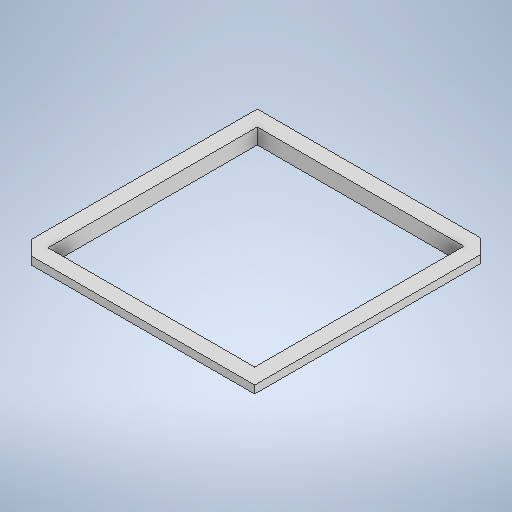
# Autodesk Inventor part: Installation Tool Collar
Saved by Autodesk Inventor 2025 (Build 290162000, 162)
## iProperties
Created: 2025-03-25
Part Number: Installation Tool Collar
Material: Generic
Document SubType Name: Modeling
Designer: Caleb Fangmeier
Density: 1 g/cm^3
Appearance: Default
Author: Caleb Fangmeier
Autodesk Inventor part; units mm, degrees
ref_plane "YZ Plane" through (0, 0, 0) normal (1, 0, 0) x (0, 1, 0)
ref_plane "XZ Plane" through (0, 0, 0) normal (0, 1, 0) x (-1, 0, 0)
ref_plane "XY Plane" through (0, 0, 0) normal (0, 0, 1) x (1, 0, 0)
sketch "Sketch1" plane through (0, 0, 0) normal (0, 1, 0) x (-1, 0, 0)
  line L0 (-21.4, -21.65) -> (21.4, -21.65)
  line L1 (21.4, -21.65) -> (21.4, 21.65)
  line L2 (21.4, 21.65) -> (-21.4, 21.65)
  line L3 (-21.4, 21.65) -> (-21.4, -21.65)
  line L4 (-21.4, -21.65) -> (21.4, 21.65) construction
  line L5 (21.4, -21.65) -> (-21.4, 21.65) construction
  point P0 (0, 0)
  dimension "d0" = 43.3
  dimension "d1" = 42.8
  constraints: 12 end point, 2 midpoint, 2 parallel, 1 horizontal, 1 perpendicular
  measures "d0" distance of L0.end L1.end
  measures "d1" distance of L0.start L0.end
extrude "Extrusion1" add sketch "Sketch1" along normal blind 1.5
sketch "Sketch2" plane through (0, 1.5, 0) normal (0, 1, 0) x (1, 0, 0)
  line L0 (22.9, 23.15) -> (-22.9, 23.15)
  line L1 (-22.9, 23.15) -> (-22.9, -23.15)
  line L2 (-22.9, -23.15) -> (22.9, -23.15)
  line L3 (22.9, -23.15) -> (22.9, 23.15)
  line L4 (22.9, 23.15) -> (-22.9, -23.15) construction
  line L5 (-22.9, 23.15) -> (22.9, -23.15) construction
  line L6 (-21.4, 21.65) -> (-21.4, -21.65) projected
  line L7 (-21.4, -21.65) -> (21.4, -21.65) projected
  point P0 (0, 0)
  dimension "d4" = 1.5
  dimension "d5" = 1.5
  constraints: 12 end point, 2 midpoint, 2 parallel, 1 horizontal, 1 perpendicular
  measures "d4" distance between parallel lines of L1 L6
  measures "d5" distance between parallel lines of L2 L7
extrude "Extrusion2" add sketch "Sketch2" along normal blind 1.5
sketch "Sketch3" plane through (0, 3, 0) normal (0, 1, 0) x (1, 0, 0)
  line L0 (19.9, 20.15) -> (-19.9, 20.15)
  line L1 (-19.9, 20.15) -> (-19.9, -20.15)
  line L2 (-19.9, -20.15) -> (19.9, -20.15)
  line L3 (19.9, -20.15) -> (19.9, 20.15)
  line L4 (19.9, 20.15) -> (-19.9, -20.15) construction
  line L5 (-19.9, 20.15) -> (19.9, -20.15) construction
  line L6 (-21.4, -21.65) -> (21.4, -21.65) projected
  line L7 (-21.4, 21.65) -> (-21.4, -21.65) projected
  point P0 (0, 0)
  dimension "d8" = 1.5
  dimension "d9" = 1.5
  constraints: 12 end point, 2 midpoint, 2 parallel, 1 horizontal, 1 perpendicular
  measures "d8" distance between parallel lines of L6 L2
  measures "d9" distance between parallel lines of L7 L1
extrude "Extrusion3" cut sketch "Sketch3" against normal through all
chamfer "Chamfer1" distance 2.9 angle 45 2 edges at (22.9, 2.25, -23.15) (-22.9, 2.25, 23.15)
sketch "Sketch4" plane through (21.4, 0, 21.65) normal (1, 0, 0) x (0, 0, -1)
  line L0 (1.4, 1.5) -> (-1.5, 1.5) projected
  line L1 (-0.75, 1.5) -> (44.05, 1.5)
  line L2 (44.05, 1.5) -> (44.05, 0)
  line L3 (44.05, 0) -> (-0.75, 0)
  line L4 (-0.75, 0) -> (-0.75, 1.5)
  line L5 (0, 0) -> (43.3, 0) projected
  line L6 (-0.75, 0.75) -> (0, 0)
  line L7 (-0.75, 0.75) -> (0, 1.5)
  line L8 (21.65, 9.7528) -> (21.65, -18.8519)
  line L9 (0, 0) -> (0, 1.5) projected
  line L10 (44.05, 0.75) -> (43.3, 0)
  line L11 (44.05, 0.75) -> (43.3, 1.5)
  line L12 (43.3, 0) -> (43.3, 1.5)
  point P0 (21.65, 0)
  point P1 (21.65, 0)
  point P2 (21.65, 0)
  dimension "d16" = 44.8
  dimension "d17" = 22.4
  dimension "d18" = 0.75
  constraints: 20 end point, 5 point on line, 4 symmetric about line, 3 midpoint, 2 parallel, 1 horizontal, 1 perpendicular, 1 vertical, 1 vertical alignment
  measures "d16" distance of L2.end L3.end
  measures "d17" distance from line of L4 point (21.65, 0)
  measures "d18" horizontal distance of L6.end L6.start
extrude "Extrusion4" add sketch "Sketch4" against normal up to surface (42.8 mm away) contours L9 L6 L7 | L11 L10 L12
chamfer "Chamfer2" distance 0.5 angle 45 8 edges at (-21.4, 0.375, -22.025) (-21.4, 1.125, -22.025) (-21.4, 0.375, 22.025) (-21.4, 1.125, 22.025) (21.4, 0.375, 22.025) (21.4, 1.125, 22.025) (21.4, 0.375, -22.025) (21.4, 1.125, -22.025)
equation "\"d17\" = 0.5 * d16"
body "Solid1"
